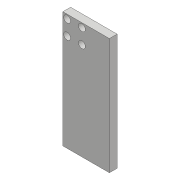
# Autodesk Inventor part: Battery_Cover
Saved by Autodesk Inventor 2018 (Build 220112000, 112)
## iProperties
Created: 2019-09-17
Part Number: Battery_Cover
Material: Generic
Document SubType Name: Modeling
Designer: Clevo
Density: 1 g/cm^3
Appearance: Default
Author: Clevo
Autodesk Inventor part; units mm, degrees
ref_plane "YZ Plane" through (0, 0, 0) normal (1, 0, 0) x (0, 1, 0)
ref_plane "XZ Plane" through (0, 0, 0) normal (0, 1, 0) x (-1, 0, 0)
ref_plane "XY Plane" through (0, 0, 0) normal (0, 0, 1) x (1, 0, 0)
sketch "Sketch1" plane through (0, 0, 0) normal (0, 1, 0) x (-1, 0, 0)
  line L0 (-22, -55) -> (22, -55)
  line L1 (22, -55) -> (22, 55)
  line L2 (22, 55) -> (-22, 55)
  line L3 (-22, 55) -> (-22, -55)
  line L4 (-22, -55) -> (22, 55) construction
  line L5 (22, -55) -> (-22, 55) construction
  point P0 (0, 0)
  dimension "d0" = 110
  dimension "d1" = 44
  constraints: 12 end point, 2 midpoint, 2 parallel, 1 horizontal, 1 perpendicular
  measures "d0" distance of L0.end L1.end
  measures "d1" distance of L1.end L2.end
extrude "Extrusion1" add sketch "Sketch1" along normal blind 7.3
sketch "Sketch2" plane through (0, 7.3, 0) normal (0, 1, 0) x (1, 0, 0)
  line L0 (22, 55) -> (-22, 55) projected
  line L1 (-22, 55) -> (-22, -55) projected
  line L2 (-22, -55) -> (22, -55) projected
  line L3 (22, -55) -> (22, 55) projected
  line L4 (0, -33) -> (-22, -33)
  line L5 (-22, -33) -> (-22, -55)
  line L6 (-22, -55) -> (0, -55)
  line L7 (0, -55) -> (0, -33)
  line L8 (0, -33) -> (-22, -55) construction
  line L9 (-22, -33) -> (0, -55) construction
  line L10 (-4, -37) -> (-18, -37)
  line L11 (-18, -37) -> (-18, -51)
  line L12 (-18, -51) -> (-4, -51)
  line L13 (-4, -51) -> (-4, -37)
  line L14 (-4, -37) -> (-18, -51) construction
  line L15 (-18, -37) -> (-4, -51) construction
  circle A0 centre (-18, -51) radius 3.25
  line L16 (-22, 55) -> (-22, -55) projected
  circle A1 centre (-18, -37) radius 3.25
  circle A2 centre (-4, -51) radius 3.25
  circle A3 centre (-4, -37) radius 3.25
  circle A4 centre (-11, -44) radius 3.75
  point P0 (0, 0)
  dimension "d4" = 22
  dimension "d5" = 22
  dimension "d6" = 14
  dimension "d7" = 7.5
  dimension "d12" = 6.5
  dimension "d13" = 6.5
  dimension "d14" = 6.5
  dimension "d15" = 6.5
  constraints: 24 end point, 5 centre point, 5 coincident, 4 midpoint, 4 parallel, 2 horizontal, 2 perpendicular, 1 point on line
  measures "d4" distance of L4.start L4.end
  measures "d5" distance of L6.end L4.start
  measures "d6" distance of L11.end L12.end
  measures "d7" diameter of A4
  measures "d12" diameter of A0
  measures "d13" diameter of A1
  measures "d14" diameter of A3
  measures "d15" diameter of A2
extrude "Extrusion2" cut sketch "Sketch2" against normal blind 6.7 contours A1 L11 L10 | L10 L11 A1 | A3 L13 L10 | L10 L13 A3 | A0 L12 L11 | L11 L12 A0 | A2 L12 L13 | L13 L12 A2 | A4
sketch "Sketch3" plane through (0, 0.6, 0) normal (0, 1, 0) x (1, 0, 0)
  circle A0 centre (-18, -51) radius 3.25 projected
  circle A1 centre (-18, -37) radius 3.25 projected
  circle A2 centre (-4, -51) radius 3.25 projected
  circle A3 centre (-4, -37) radius 3.25 projected
  point P0 (0, 0)
extrude "Extrusion3" cut sketch "Sketch3" against normal through all
equation "\"d5\" = d4"
equation "\"d13\" = d12"
equation "\"d14\" = d13"
equation "\"d15\" = d14"
body "Solid1"
